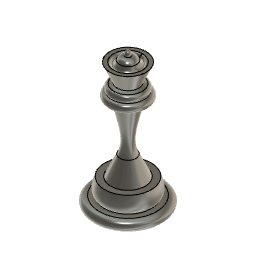
chess piece 2 v4 (Autodesk Fusion 360 design; units mm, degrees)
Autodesk Fusion 360 part; units mm, degrees
sketch "Sketch1" plane through (0, 0, 0) normal (1, 0, 0) x (0, 1, 0)
  line L0 (0, -13) -> (0, 15)
  line L1 (0, -13) -> (5.5, -13)
  spline S0 degree 5 poles (5.5, -13) (5.5818, -13) (5.7377, -12.9886) (5.9483, -12.9372) (6.182, -12.8054) (6.3897, -12.5642) (6.5061, -12.2828) (6.525, -11.9977) (6.4455, -11.7391) (6.2771, -11.5237) (6.0342, -11.3593) (5.7918, -11.2708) (5.588, -11.2287) (5.4429, -11.2114) (5.3681, -11.2054) knots 0 0 0 0 0 0 0.1 0.2 0.3 0.4 0.5 0.6 0.7 0.8 0.9 1 1 1 1 1 1
  arc A0 (5.3681, -11.2054) -> (4.3622, -11.2181) centre (4.9335, -16.6382) ccw
  spline S1 degree 5 poles (4.3622, -11.2181) (4.4013, -11.1795) (4.4761, -11.1003) (4.5777, -10.9753) (4.6915, -10.7963) (4.7957, -10.5506) (4.8585, -10.281) (4.8774, -9.9862) (4.852, -9.6658) (4.7851, -9.3215) (4.6804, -8.9555) (4.5691, -8.6468) (4.4712, -8.4069) (4.3995, -8.2433) (4.3622, -8.1607) knots 0 0 0 0 0 0 0.1 0.2 0.3 0.4 0.5 0.6 0.7 0.8 0.9 1 1 1 1 1 1
  line L2 (3.229, -8.1607) -> (4.3622, -8.1607)
  line L3 (1.5, -4.5) -> (3.229, -8.1607)
  spline S2 degree 5 poles (1.5, -4.5) (1.4082, -4.3056) (1.247, -3.9111) (1.0723, -3.3022) (0.9663, -2.4606) (1.0028, -1.3859) (1.1557, -0.3231) (1.3709, 0.6918) (1.6008, 1.627) (1.8127, 2.464) (1.991, 3.1993) (2.102, 3.7081) (2.1673, 4.047) (2.203, 4.2543) (2.2189, 4.3533) knots 0 0 0 0 0 0 0.1 0.2 0.3 0.4 0.5 0.6 0.7 0.8 0.9 1 1 1 1 1 1
  line L4 (2.2189, 4.3533) -> (3, 4.3533)
  arc A1 (3, 4.3533) -> (3, 5.8107) centre (3, 5.082) ccw
  arc A2 (3, 5.8107) -> (2.6515, 6.9837) centre (2.5013, 6.3008) ccw
  arc A3 (2.004, 7.1683) -> (2.6515, 6.9837) centre (3.8298, 12.3443) ccw
  line L5 (3.3911, 10.4454) -> (2.004, 7.1683)
  line L6 (3.3911, 10.4454) -> (2.6975, 10.4454)
  spline S3 degree 5 poles (2.6975, 10.4454) (2.6544, 10.4454) (2.5749, 10.4383) (2.4758, 10.4065) (2.38, 10.3279) (2.2995, 10.2043) (2.233, 10.0972) (2.1577, 10.0453) (2.0605, 10.0717) (1.9431, 10.1752) (1.8151, 10.3418) (1.7147, 10.5106) (1.6457, 10.6497) (1.6033, 10.7469) (1.583, 10.7966) knots 0 0 0 0 0 0 0.1 0.2 0.3 0.4 0.5 0.6 0.7 0.8 0.9 1 1 1 1 1 1
  arc A4 (1.583, 10.7966) -> (0.5, 11.5) centre (0.5354, 10.369) ccw
  arc A5 (0.5, 11.5) -> (0, 12.4015) centre (-0.1818, 11.7112) ccw
  point P0 (6.5, -12)
  point P1 (4.8648, -10.0849)
  point P2 (1.5, 1.208)
  point P3 (2.1684, 10.0682)
  constraint vertical L0
  constraint perpendicular L0 L1
  constraint tangent S0 A0
  constraint horizontal L2
  constraint horizontal L4
  constraint tangent L4 A1
  constraint tangent A2 A3
  constraint horizontal L6
  constraint tangent S3 A4
  constraint coincident L0 A5.end
revolve "Revolve1" add sketch "Sketch1" angle 360 about axis through (0, 0, -13) along (0, 0, 1)
